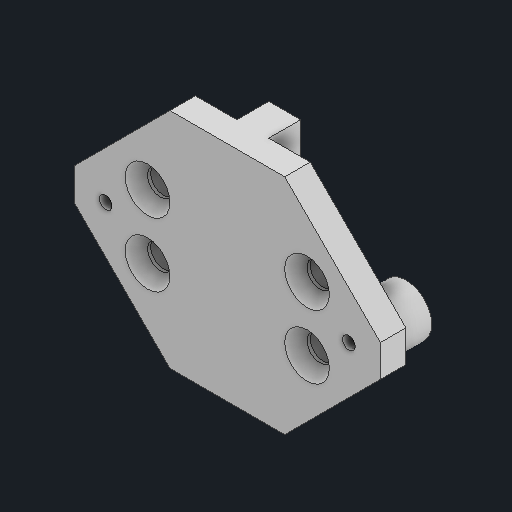
# Autodesk Inventor part: Base
Saved by Autodesk Inventor 2026.1 (Build 301233000, 233)
## iProperties
Created: 2026-05-05
Part Number: Base
Material: Generic
Document SubType Name: Modeling
Designer: aleja
Density: 1 g/cm^3
Appearance: Default
Author: aleja
Autodesk Inventor part; units mm, degrees
ref_plane "YZ Plane" through (0, 0, 0) normal (1, 0, 0) x (0, 1, 0)
ref_plane "XZ Plane" through (0, 0, 0) normal (0, 1, 0) x (-1, 0, 0)
ref_plane "XY Plane" through (0, 0, 0) normal (0, 0, 1) x (1, 0, 0)
sketch "Sketch1" plane through (0, 0, 0) normal (0, 1, 0) x (-1, 0, 0)
  line L0 (-24, 17.5) -> (24, 17.5)
  line L1 (24, 17.5) -> (24, -17.5)
  line L2 (24, -17.5) -> (-24, -17.5)
  line L3 (-24, -17.5) -> (-24, 17.5)
  line L4 (-24, 17.5) -> (24, -17.5) construction
  line L5 (24, 17.5) -> (-24, -17.5) construction
  point P0 (0, 0)
  dimension "d0" = 48
  dimension "d1" = 35
  constraints: 12 end point, 2 midpoint, 2 parallel, 1 horizontal, 1 perpendicular
  measures "d0" distance of L1.end L2.end
  measures "d1" distance of L0.end L1.end
extrude "Extrusion1" add sketch "Sketch1" along normal blind 4
sketch "Sketch2" plane through (0, 4, 0) normal (0, 1, 0) x (1, 0, 0)
  line L0 (0, 0) -> (-5.2635, 0) construction
  line L1 (-5.2635, 0) -> (-5.2635, 9.5172) construction
  line L2 (-5.2635, 9.5172) -> (0, 9.5172) construction
  line L3 (0, 9.5172) -> (0, 0) construction
  circle A0 centre (-19.05, 0) radius 1
  circle A1 centre (19.05, 0) radius 1
  circle A2 centre (-19.05, 0) radius 4
  circle A3 centre (19.05, 0) radius 4
  line L4 (-24, -17.5) -> (24, -17.5) projected
  line L5 (0, -17.5) -> (-2.5, -17.5)
  line L6 (-2.5, -17.5) -> (-2.5, -12.5)
  line L7 (-2.5, -12.5) -> (0, -12.5)
  line L8 (0, -12.5) -> (0, -17.5)
  line L9 (2.5, -17.5) -> (2.5, -12.5)
  line L10 (2.5, -12.5) -> (0, -12.5)
  line L11 (-2.5, 17.5) -> (-2.5, 12.5)
  line L12 (-2.5, 12.5) -> (0, 12.5)
  line L13 (2.5, 17.5) -> (2.5, 12.5)
  line L14 (2.5, 12.5) -> (0, 12.5)
  line L15 (24, 17.5) -> (-24, 17.5) projected
  dimension "d4" = 2
  dimension "d5" = 19.05
  dimension "d6" = 3
  dimension "d7" = 3
  dimension "d8" = 2.5
  dimension "d9" = 5
  constraints: 28 end point, 8 symmetric about line, 4 centre point, 4 parallel, 2 horizontal, 2 perpendicular, 1 midpoint, 1 point on line, 1 other
  measures "d4" diameter of A0
  measures "d5" distance from line of L3 A0.centre
  measures "d6" radial gap between concentric circles of A0 A2
  measures "d7" radial gap between concentric circles of A1 A3
  measures "d8" distance of L6.end L7.end
  measures "d9" distance of L5.end L6.end
extrude "Extrusion2" add sketch "Sketch2" along normal blind 5
chamfer "Chamfer1" distance 15 angle 45 4 edges at (24, 2, -17.5) (24, 2, 17.5) (-24, 2, 17.5) (-24, 2, -17.5)
sketch "Sketch4" plane through (19.05, 9, 0) normal (0, 1, 0) x (1, 0, 0)
  circle A0 centre (0, 0) radius 1 projected
  circle A1 centre (-38.1, 0) radius 1 projected
  point P0 (-19.05, 0)
extrude "Extrusion3" cut sketch "Sketch4" against normal through all
sketch "Sketch7" plane through (0, 0, 0) normal (0, -1, 0) x (1, 0, 0)
  line L0 (14.5, -3) -> (10.5, -3)
  line L1 (10.5, -3) -> (10.5, -7)
  line L2 (10.5, -7) -> (14.5, -7)
  line L3 (14.5, -7) -> (14.5, -3)
  line L4 (0, -6.5734) -> (0, 0) construction
  line L5 (0, 0) -> (6.1677, 0) construction
  line L6 (-14.5, -3) -> (-10.5, -3)
  line L7 (-10.5, -3) -> (-10.5, -7)
  line L8 (-10.5, -7) -> (-14.5, -7)
  line L9 (-14.5, -7) -> (-14.5, -3)
  line L10 (14.5, 3) -> (10.5, 3)
  line L11 (10.5, 3) -> (10.5, 7)
  line L12 (10.5, 7) -> (14.5, 7)
  line L13 (14.5, 7) -> (14.5, 3)
  line L14 (-10.5, 7) -> (-14.5, 7)
  line L15 (-10.5, 3) -> (-10.5, 7)
  line L16 (-14.5, 3) -> (-10.5, 3)
  line L17 (-14.5, 7) -> (-14.5, 3)
  circle A0 centre (12.5, -5) radius 2
  circle A1 centre (-12.5, -5) radius 2
  circle A2 centre (12.5, 5) radius 2
  circle A3 centre (-12.5, 5) radius 2
  point P0 (12.5, -7)
  point P1 (10.5, -5)
  point P2 (12.5, 7)
  point P3 (10.5, 5)
  point P4 (12.5, -3)
  dimension "d30" = 12.5
  dimension "d31" = 4
  dimension "d32" = 4
  dimension "d33" = 5
  constraints: 36 end point, 17 symmetric about line, 4 centre point, 3 midpoint, 3 point on circle, 2 horizontal, 2 parallel, 1 perpendicular, 3 other
  measures "d30" horizontal distance of L4.end A0.start
  measures "d31" distance of L1.end L2.end
  measures "d32" distance of L2.end L0.start
  measures "d33" vertical distance of L4.end point (10.5, -5)
extrude "Extrusion6" cut sketch "Sketch7" against normal blind 2.5 contours A0 | A1 | A2 | A3
chamfer "Chamfer3" distance 1.5 distance2 2 4 edges at (10.5, 0, 5) (10.5, 0, -5) (-14.5, 0, -5) (-14.5, 0, 5) measured on face at (3, 0, -9.7863)
chamfer "Chamfer4" distance 2 angle 45 2 edges at (-20.05, 9, 0) (18.05, 9, 0)
equation "\"d32\" = d31"
body "Solid1"
